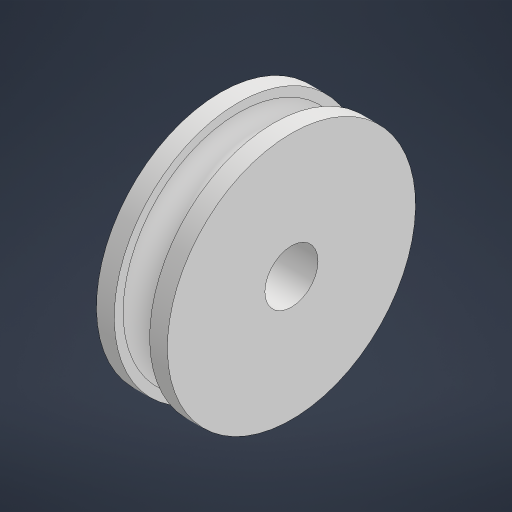
# Autodesk Inventor part: Pulley_Big
Saved by Autodesk Inventor 2024.2 (Build 282272000, 272)
## iProperties
Created: 2024-01-10
Part Number: Pulley_Big
Material: 一般
Document SubType Name: Modeling
Designer: Hanaoka
Density: 1 g/cm^3
Appearance: 既定
Author: Hanaoka
Autodesk Inventor part; units mm, degrees
ref_plane "YZ Plane" through (0, 0, 0) normal (1, 0, 0) x (0, 1, 0)
ref_plane "XZ Plane" through (0, 0, 0) normal (0, 1, 0) x (-1, 0, 0)
ref_plane "XY Plane" through (0, 0, 0) normal (0, 0, 1) x (1, 0, 0)
sketch "スケッチ1" plane through (0, 0, 0) normal (0, 0, 1) x (1, 0, 0)
  line L0 (-2, 7) -> (-2, 1.5)
  line L1 (-2, 1.5) -> (2, 1.5)
  line L2 (2, 1.5) -> (2, 7)
  line L3 (-2, 7) -> (-1, 7)
  line L4 (2, 7) -> (1, 7)
  line L5 (1, 7) -> (1, 6.5)
  line L6 (-1, 7) -> (-1, 6.5)
  arc A0 (-1, 6.5) -> (1, 6.5) centre (0, 6.5) ccw
  line L7 (0, 6.5) -> (0, 1.5) construction
  line L8 (0, -1.4) -> (0, 8.4) projected
  line L9 (-2.8, 0) -> (2.8, 0) projected
  point P0 (0, 0)
  dimension "d0" = 1.5
  dimension "d1" = 7
  dimension "d2" = 1
  dimension "d3" = 1
  dimension "d4" = 0.5
  constraints: 16 end point, 3 perpendicular, 2 equal length, 2 point on circle, 2 point on line, 2 vertical, 1 centre point, 1 horizontal, 1 midpoint, 1 parallel, 1 tangent
  measures "d0" distance from line of point (0, 0) L1
  measures "d1" vertical distance of point (0, 0) L0.start
  measures "d2" distance of L2.end L4.end
  measures "d3" radius of A0
  measures "d4" distance of L4.end L5.end
revolve "回転1" add sketch "スケッチ1" angle 360 about axis through (-10, 0, 0) along (1, 0, 0)
